Autodesk Inventor part; units mm, degrees
(part 3 of 3)
  line L321 (6.6942, 97.0319) -> (-7.3058, 97.0327) projected
  line L322 (16.4442, 97.0314) -> (16.445, 110.9522) projected
  line L323 (16.445, 110.9522) -> (30.445, 110.9515) projected
  line L324 (30.445, 110.9515) -> (30.4442, 97.0307) projected
  line L325 (30.4442, 97.0307) -> (16.4442, 97.0314) projected
  line L326 (6.9432, 78.1394) -> (6.944, 92.0602) projected
  line L327 (6.944, 92.0602) -> (20.944, 92.0594) projected
  line L328 (20.944, 92.0594) -> (20.9432, 78.1386) projected
  line L329 (20.9432, 78.1386) -> (6.9432, 78.1394) projected
  line L330 (11.6922, 59.2466) -> (11.693, 73.1674) projected
  line L331 (11.693, 73.1674) -> (25.693, 73.1667) projected
  line L332 (25.693, 73.1667) -> (25.6922, 59.2458) projected
  line L333 (25.6922, 59.2458) -> (11.6922, 59.2466) projected
  line L334 (14.0662, 40.3539) -> (14.067, 54.2747) projected
  line L335 (14.067, 54.2747) -> (28.067, 54.274) projected
  line L336 (28.067, 54.274) -> (28.0662, 40.3532) projected
  line L337 (28.0662, 40.3532) -> (14.0662, 40.3539) projected
  line L338 (-209.1848, 21.4733) -> (-209.1841, 35.3941) projected
  line L339 (-209.1841, 35.3941) -> (-195.1841, 35.3934) projected
  line L340 (-195.1841, 35.3934) -> (-195.1848, 21.4726) projected
  line L341 (-195.1848, 21.4726) -> (-209.1848, 21.4733) projected
  line L342 (-190.1848, 21.4723) -> (-190.1841, 35.3931) projected
  line L343 (-190.1841, 35.3931) -> (-176.1841, 35.3924) projected
  line L344 (-176.1841, 35.3924) -> (-176.1848, 21.4716) projected
  line L345 (-176.1848, 21.4716) -> (-190.1848, 21.4723) projected
  line L346 (-171.1848, 21.4713) -> (-171.1841, 35.3921) projected
  line L347 (-171.1841, 35.3921) -> (-157.1841, 35.3914) projected
  line L348 (-157.1841, 35.3914) -> (-157.1848, 21.4705) projected
  line L349 (-157.1848, 21.4705) -> (-171.1848, 21.4713) projected
  line L350 (-152.1848, 21.4703) -> (-152.1841, 35.3911) projected
  line L351 (-152.1841, 35.3911) -> (-138.1841, 35.3903) projected
  line L352 (-138.1841, 35.3903) -> (-138.1848, 21.4695) projected
  line L353 (-138.1848, 21.4695) -> (-152.1848, 21.4703) projected
  line L354 (-133.1848, 21.4693) -> (-133.1841, 35.3901) projected
  line L355 (-133.1841, 35.3901) -> (-119.1841, 35.3893) projected
  line L356 (-119.1841, 35.3893) -> (-119.1848, 21.4685) projected
  line L357 (-119.1848, 21.4685) -> (-133.1848, 21.4693) projected
  line L358 (-114.1848, 21.4682) -> (-114.1841, 35.3891) projected
  line L359 (-114.1841, 35.3891) -> (-100.1841, 35.3883) projected
  line L360 (-100.1841, 35.3883) -> (-100.1848, 21.4675) projected
  line L361 (-100.1848, 21.4675) -> (-114.1848, 21.4682) projected
  line L362 (-95.1848, 21.4672) -> (-95.1841, 35.388) projected
  line L363 (-95.1841, 35.388) -> (-81.1841, 35.3873) projected
  line L364 (-81.1841, 35.3873) -> (-81.1848, 21.4665) projected
  line L365 (-81.1848, 21.4665) -> (-95.1848, 21.4672) projected
  line L366 (-76.1848, 21.4662) -> (-76.1841, 35.387) projected
  line L367 (-76.1841, 35.387) -> (-62.1841, 35.3863) projected
  line L368 (-62.1841, 35.3863) -> (-62.1848, 21.4655) projected
  line L369 (-62.1848, 21.4655) -> (-76.1848, 21.4662) projected
  line L370 (-57.1848, 21.4652) -> (-57.1841, 35.386) projected
  line L371 (-57.1841, 35.386) -> (-43.1841, 35.3853) projected
  line L372 (-43.1841, 35.3853) -> (-43.1848, 21.4645) projected
  line L373 (-43.1848, 21.4645) -> (-57.1848, 21.4652) projected
  line L374 (-38.1848, 21.4642) -> (-38.1841, 35.385) projected
  line L375 (-38.1841, 35.385) -> (-24.1841, 35.3843) projected
  line L376 (-24.1841, 35.3843) -> (-24.1848, 21.4634) projected
  line L377 (-24.1848, 21.4634) -> (-38.1848, 21.4642) projected
  line L378 (-19.1848, 21.4632) -> (-19.1841, 35.384) projected
  line L379 (-19.1841, 35.384) -> (-5.1841, 35.3832) projected
  line L380 (-5.1841, 35.3832) -> (-5.1848, 21.4624) projected
  line L381 (-5.1848, 21.4624) -> (-19.1848, 21.4632) projected
  line L382 (-0.1848, 21.4622) -> (-0.1841, 35.383) projected
  line L383 (-0.1841, 35.383) -> (13.8159, 35.3822) projected
  line L384 (13.8159, 35.3822) -> (13.8152, 21.4614) projected
  line L385 (13.8152, 21.4614) -> (-0.1848, 21.4622) projected
  line L386 (18.8152, 21.4611) -> (18.8159, 35.382) projected
  line L387 (18.8159, 35.382) -> (32.8159, 35.3812) projected
  line L388 (32.8159, 35.3812) -> (32.8152, 21.4604) projected
  line L389 (32.8152, 21.4604) -> (18.8152, 21.4611) projected
  line L390 (56.567, 54.2725) -> (56.5662, 40.3517) projected
  line L391 (56.5662, 40.3517) -> (42.5662, 40.3524) projected
  line L392 (42.5662, 40.3524) -> (42.567, 54.2732) projected
  line L393 (42.567, 54.2732) -> (56.567, 54.2725) projected
  line L394 (75.567, 54.2715) -> (75.5662, 40.3506) projected
  line L395 (75.5662, 40.3506) -> (61.5662, 40.3514) projected
  line L396 (61.5662, 40.3514) -> (61.567, 54.2722) projected
  line L397 (61.567, 54.2722) -> (75.567, 54.2715) projected
  line L398 (94.567, 54.2704) -> (94.5662, 40.3496) projected
  line L399 (94.5662, 40.3496) -> (80.5662, 40.3504) projected
  line L400 (80.5662, 40.3504) -> (80.567, 54.2712) projected
  line L401 (80.567, 54.2712) -> (94.567, 54.2704) projected
  line L402 (56.5659, 35.3799) -> (56.5652, 21.4591) projected
  line L403 (56.5652, 21.4591) -> (42.5652, 21.4599) projected
  line L404 (42.5652, 21.4599) -> (42.5659, 35.3807) projected
  line L405 (42.5659, 35.3807) -> (56.5659, 35.3799) projected
  line L406 (75.5659, 35.3789) -> (75.5652, 21.4581) projected
  line L407 (75.5652, 21.4581) -> (61.5652, 21.4589) projected
  line L408 (61.5652, 21.4589) -> (61.5659, 35.3797) projected
  line L409 (61.5659, 35.3797) -> (75.5659, 35.3789) projected
  line L410 (80.5652, 21.4578) -> (80.5659, 35.3787) projected
  line L411 (80.5659, 35.3787) -> (94.5659, 35.3779) projected
  line L412 (94.5659, 35.3779) -> (94.5652, 21.4571) projected
  line L413 (94.5652, 21.4571) -> (80.5652, 21.4578) projected
  line L414 (61.5682, 78.1365) -> (61.569, 92.0573) projected
  line L415 (61.569, 92.0573) -> (75.569, 92.0565) projected
  line L416 (75.569, 92.0565) -> (75.5682, 78.1357) projected
  line L417 (75.5682, 78.1357) -> (61.5682, 78.1365) projected
  line L418 (42.5692, 97.03) -> (42.57, 110.9508) projected
  line L419 (42.57, 110.9508) -> (56.57, 110.9501) projected
  line L420 (56.57, 110.9501) -> (56.5692, 97.0293) projected
  line L421 (56.5692, 97.0293) -> (42.5692, 97.03) projected
  line L422 (61.5692, 97.029) -> (61.57, 110.9498) projected
  line L423 (61.57, 110.9498) -> (75.57, 110.9491) projected
  line L424 (75.57, 110.9491) -> (75.5692, 97.0282) projected
  line L425 (75.5692, 97.0282) -> (61.5692, 97.029) projected
  line L426 (80.5692, 97.028) -> (80.57, 110.9488) projected
  line L427 (80.57, 110.9488) -> (94.57, 110.948) projected
  line L428 (94.57, 110.948) -> (94.5692, 97.0272) projected
  line L429 (94.5692, 97.0272) -> (80.5692, 97.028) projected
  line L430 (104.3187, 87.5804) -> (104.3195, 101.5013) projected
  line L431 (104.3195, 101.5013) -> (118.3195, 101.5005) projected
  line L432 (118.3195, 101.5005) -> (118.3187, 87.5797) projected
  line L433 (118.3187, 87.5797) -> (104.3187, 87.5804) projected
  line L434 (104.3167, 49.7954) -> (104.3175, 63.7162) projected
  line L435 (104.3175, 63.7162) -> (118.3175, 63.7154) projected
  line L436 (118.3175, 63.7154) -> (118.3167, 49.7946) projected
  line L437 (118.3167, 49.7946) -> (104.3167, 49.7954) projected
  line L438 (104.3152, 21.4566) -> (104.3159, 35.3774) projected
  line L439 (104.3159, 35.3774) -> (118.3159, 35.3766) projected
  line L440 (118.3159, 35.3766) -> (118.3152, 21.4558) projected
  line L441 (118.3152, 21.4558) -> (104.3152, 21.4566) projected
  line L442 (137.3192, 97.0249) -> (123.3192, 97.0257) projected
  line L443 (123.3192, 97.0257) -> (123.32, 110.9465) projected
  line L444 (123.32, 110.9465) -> (137.32, 110.9458) projected
  line L445 (137.32, 110.9458) -> (137.3192, 97.0249) projected
  line L446 (156.3192, 97.0239) -> (142.3192, 97.0247) projected
  line L447 (142.3192, 97.0247) -> (142.32, 110.9455) projected
  line L448 (142.32, 110.9455) -> (156.32, 110.9447) projected
  line L449 (156.32, 110.9447) -> (156.3192, 97.0239) projected
  line L450 (175.3192, 97.0229) -> (161.3192, 97.0237) projected
  line L451 (161.3192, 97.0237) -> (161.32, 110.9445) projected
  line L452 (161.32, 110.9445) -> (175.32, 110.9437) projected
  line L453 (175.32, 110.9437) -> (175.3192, 97.0229) projected
  line L454 (137.3182, 78.1324) -> (123.3182, 78.1332) projected
  line L455 (123.3182, 78.1332) -> (123.319, 92.054) projected
  line L456 (123.319, 92.054) -> (137.319, 92.0532) projected
  line L457 (137.319, 92.0532) -> (137.3182, 78.1324) projected
  line L458 (156.3182, 78.1314) -> (142.3182, 78.1321) projected
  line L459 (142.3182, 78.1321) -> (142.319, 92.053) projected
  line L460 (142.319, 92.053) -> (156.319, 92.0522) projected
  line L461 (156.319, 92.0522) -> (156.3182, 78.1314) projected
  line L462 (175.3182, 78.1304) -> (161.3182, 78.1311) projected
  line L463 (161.3182, 78.1311) -> (161.319, 92.0519) projected
  line L464 (161.319, 92.0519) -> (175.319, 92.0512) projected
  line L465 (175.319, 92.0512) -> (175.3182, 78.1304) projected
  line L466 (137.3172, 59.2399) -> (123.3172, 59.2406) projected
  line L467 (123.3172, 59.2406) -> (123.318, 73.1614) projected
  line L468 (123.318, 73.1614) -> (137.318, 73.1607) projected
  line L469 (137.318, 73.1607) -> (137.3172, 59.2399) projected
  line L470 (156.3172, 59.2389) -> (142.3172, 59.2396) projected
  line L471 (142.3172, 59.2396) -> (142.318, 73.1604) projected
  line L472 (142.318, 73.1604) -> (156.318, 73.1597) projected
  line L473 (156.318, 73.1597) -> (156.3172, 59.2389) projected
  line L474 (175.3172, 59.2379) -> (161.3172, 59.2386) projected
  line L475 (161.3172, 59.2386) -> (161.318, 73.1594) projected
  line L476 (161.318, 73.1594) -> (175.318, 73.1587) projected
  line L477 (175.318, 73.1587) -> (175.3172, 59.2379) projected
  line L478 (137.3162, 40.3474) -> (123.3162, 40.3481) projected
  line L479 (123.3162, 40.3481) -> (123.317, 54.2689) projected
  line L480 (123.317, 54.2689) -> (137.317, 54.2682) projected
  line L481 (137.317, 54.2682) -> (137.3162, 40.3474) projected
  line L482 (156.3162, 40.3463) -> (142.3162, 40.3471) projected
  line L483 (142.3162, 40.3471) -> (142.317, 54.2679) projected
  line L484 (142.317, 54.2679) -> (156.317, 54.2671) projected
  line L485 (156.317, 54.2671) -> (156.3162, 40.3463) projected
  line L486 (175.3162, 40.3453) -> (161.3162, 40.3461) projected
  line L487 (161.3162, 40.3461) -> (161.317, 54.2669) projected
  line L488 (161.317, 54.2669) -> (175.317, 54.2661) projected
  line L489 (175.317, 54.2661) -> (175.3162, 40.3453) projected
  line L490 (137.3152, 21.4548) -> (123.3152, 21.4556) projected
  line L491 (123.3152, 21.4556) -> (123.3159, 35.3764) projected
  line L492 (123.3159, 35.3764) -> (137.3159, 35.3756) projected
  line L493 (137.3159, 35.3756) -> (137.3152, 21.4548) projected
  line L494 (156.3152, 21.4538) -> (142.3152, 21.4546) projected
  line L495 (142.3152, 21.4546) -> (142.3159, 35.3754) projected
  line L496 (142.3159, 35.3754) -> (156.3159, 35.3746) projected
  line L497 (156.3159, 35.3746) -> (156.3152, 21.4538) projected
  line L498 (161.3152, 21.4535) -> (161.3159, 35.3743) projected
  line L499 (161.3159, 35.3743) -> (175.3159, 35.3736) projected
  line L500 (175.3159, 35.3736) -> (175.3152, 21.4528) projected
  line L501 (175.3152, 21.4528) -> (161.3152, 21.4535) projected
  line L502 (-247.1863, -6.8635) -> (-247.1856, 7.0574) projected
  line L503 (-247.1856, 7.0574) -> (-233.1856, 7.0566) projected
  line L504 (-233.1856, 7.0566) -> (-233.1863, -6.8642) projected
  line L505 (-233.1863, -6.8642) -> (-247.1863, -6.8635) projected
  line L506 (-228.1863, -6.8645) -> (-228.1856, 7.0563) projected
  line L507 (-228.1856, 7.0563) -> (-214.1856, 7.0556) projected
  line L508 (-214.1856, 7.0556) -> (-214.1863, -6.8652) projected
  line L509 (-214.1863, -6.8652) -> (-228.1863, -6.8645) projected
  line L510 (-209.1863, -6.8655) -> (-209.1856, 7.0553) projected
  line L511 (-209.1856, 7.0553) -> (-195.1856, 7.0546) projected
  line L512 (-195.1856, 7.0546) -> (-195.1863, -6.8662) projected
  line L513 (-195.1863, -6.8662) -> (-209.1863, -6.8655) projected
  line L514 (-190.1863, -6.8665) -> (-190.1856, 7.0543) projected
  line L515 (-190.1856, 7.0543) -> (-176.1856, 7.0536) projected
  line L516 (-176.1856, 7.0536) -> (-176.1863, -6.8672) projected
  line L517 (-176.1863, -6.8672) -> (-190.1863, -6.8665) projected
  line L518 (-161.6863, -6.868) -> (-161.6856, 7.0528) projected
  line L519 (-161.6856, 7.0528) -> (-147.6856, 7.052) projected
  line L520 (-147.6856, 7.052) -> (-147.6863, -6.8688) projected
  line L521 (-147.6863, -6.8688) -> (-161.6863, -6.868) projected
  line L522 (-142.6863, -6.869) -> (-142.6856, 7.0518) projected
  line L523 (-142.6856, 7.0518) -> (-128.6856, 7.051) projected
  line L524 (-128.6856, 7.051) -> (-128.6863, -6.8698) projected
  line L525 (-128.6863, -6.8698) -> (-142.6863, -6.869) projected
  line L526 (-123.6863, -6.87) -> (-123.6856, 7.0508) projected
  line L527 (-123.6856, 7.0508) -> (-109.6856, 7.05) projected
  line L528 (-109.6856, 7.05) -> (-109.6863, -6.8708) projected
  line L529 (-109.6863, -6.8708) -> (-123.6863, -6.87) projected
  line L530 (-104.6863, -6.8711) -> (-104.6856, 7.0498) projected
  line L531 (-104.6856, 7.0498) -> (-90.6856, 7.049) projected
  line L532 (-90.6856, 7.049) -> (-90.6863, -6.8718) projected
  line L533 (-90.6863, -6.8718) -> (-104.6863, -6.8711) projected
  line L534 (-76.1863, -6.8726) -> (-76.1856, 7.0482) projected
  line L535 (-76.1856, 7.0482) -> (-62.1856, 7.0475) projected
  line L536 (-62.1856, 7.0475) -> (-62.1863, -6.8733) projected
  line L537 (-62.1863, -6.8733) -> (-76.1863, -6.8726) projected
  line L538 (-57.1863, -6.8736) -> (-57.1856, 7.0472) projected
  line L539 (-57.1856, 7.0472) -> (-43.1856, 7.0465) projected
  line L540 (-43.1856, 7.0465) -> (-43.1863, -6.8743) projected
  line L541 (-43.1863, -6.8743) -> (-57.1863, -6.8736) projected
  line L542 (-38.1863, -6.8746) -> (-38.1856, 7.0462) projected
  line L543 (-38.1856, 7.0462) -> (-24.1856, 7.0455) projected
  line L544 (-24.1856, 7.0455) -> (-24.1863, -6.8754) projected
  line L545 (-24.1863, -6.8754) -> (-38.1863, -6.8746) projected
  line L546 (-19.1863, -6.8756) -> (-19.1856, 7.0452) projected
  line L547 (-19.1856, 7.0452) -> (-5.1856, 7.0444) projected
  line L548 (-5.1856, 7.0444) -> (-5.1863, -6.8764) projected
  line L549 (-5.1863, -6.8764) -> (-19.1863, -6.8756) projected
  line L550 (18.8137, -6.8777) -> (18.8144, 7.0432) projected
  line L551 (18.8144, 7.0432) -> (32.8144, 7.0424) projected
  line L552 (32.8144, 7.0424) -> (32.8137, -6.8784) projected
  line L553 (32.8137, -6.8784) -> (18.8137, -6.8777) projected
  line L554 (-252.0614, -9.3491) -> (180.1886, -9.3721) projected
  ellipse E814 centre (180.1888, -4.649) end of major axis (184.9388, -4.6493) minor radius 4.7231 (180.1886, -9.3721) -> (184.9388, -4.6493) ccw projected
  line L555 (184.9388, -4.6493) -> (184.9449, 108.7059) projected
  ellipse E815 centre (180.1949, 108.7062) end of major axis (184.9449, 108.7059) minor radius 4.7231 (184.9449, 108.7059) -> (180.1951, 113.4293) ccw projected
  line L556 (180.1951, 113.4293) -> (-252.0549, 113.4524) projected
  ellipse E816 centre (-252.0551, 108.7293) end of major axis (-256.8051, 108.7295) minor radius 4.7231 (-252.0549, 113.4524) -> (-256.8051, 108.7295) ccw projected
  line L557 (-256.8051, 108.7295) -> (-256.8112, -4.6257) projected
  ellipse E817 centre (-252.0612, -4.6259) end of major axis (-256.8112, -4.6257) minor radius 4.7231 (-256.8112, -4.6257) -> (-252.0614, -9.3491) ccw projected
  line L558 (180.1884, -12.9036) -> (-252.0616, -12.8805)
  line L559 (-259.8112, -5.157) -> (-259.8052, 108.1982)
  line L560 (-252.0548, 115.921) -> (180.1952, 115.8979)
  line L561 (187.9449, 108.1743) -> (187.9388, -5.1809)
  line L562 (187.9449, 108.7058) -> (187.9388, -4.6494)
  line L563 (180.1884, -12.3722) -> (-252.0616, -12.3491)
  line L564 (-259.8112, -4.6255) -> (-259.8052, 108.7297)
  line L565 (-252.0547, 116.4524) -> (180.1953, 116.4294)
  ellipse E818 centre (-168.9362, -4.6304) end of major axis (-167.5862, -4.6304) minor radius 1.3424 projected
  ellipse E819 centre (-223.5588, 40.2423) end of major axis (-222.2088, 40.2423) minor radius 1.3424 projected
  ellipse E820 centre (-202.181, 92.1956) end of major axis (-200.831, 92.1956) minor radius 1.3424 projected
  ellipse E821 centre (-145.1839, 38.6323) end of major axis (-143.8339, 38.6322) minor radius 1.3424 projected
  ellipse E822 centre (-111.9319, 74.9996) end of major axis (-110.5819, 74.9995) minor radius 1.3424 projected
  ellipse E823 centre (-69.1839, 38.6282) end of major axis (-67.8339, 38.6281) minor radius 1.3424 projected
  ellipse E824 centre (139.8181, 75.6464) end of major axis (141.1681, 75.6464) minor radius 1.3424 projected
  ellipse E825 centre (139.8161, 37.8614) end of major axis (141.1661, 37.8613) minor radius 1.3424 projected
  ellipse E826 centre (78.0661, 37.8647) end of major axis (79.4161, 37.8646) minor radius 1.3424 projected
  ellipse E827 centre (-83.4362, -4.6349) end of major axis (-82.0862, -4.635) minor radius 1.3424 projected
  ellipse E828 centre (-26.4319, 76.2579) end of major axis (-25.0819, 76.2578) minor radius 1.3424 projected
  ellipse E829 centre (37.6888, -4.6414) end of major axis (39.0388, -4.6415) minor radius 1.3424 projected
  ellipse E830 centre (9.1912, 40.2299) end of major axis (10.5412, 40.2298) minor radius 1.3424 projected
  ellipse E831 centre (30.5678, 70.9291) end of major axis (31.9178, 70.9291) minor radius 1.3424 projected
  ellipse E832 centre (180.1918, 52.0286) end of major axis (181.5418, 52.0285) minor radius 1.3424 projected
  ellipse E833 centre (180.1888, -4.649) end of major axis (181.5388, -4.6491) minor radius 1.3424 projected
  ellipse E834 centre (180.1949, 108.7062) end of major axis (181.5449, 108.7061) minor radius 1.3424 projected
  ellipse E835 centre (11.5699, 108.7152) end of major axis (12.9199, 108.7151) minor radius 1.3424 projected
  ellipse E836 centre (97.8229, 108.7106) end of major axis (99.1729, 108.7105) minor radius 1.3424 projected
  ellipse E837 centre (-59.6801, 108.719) end of major axis (-58.3301, 108.7189) minor radius 1.3424 projected
  ellipse E838 centre (-154.6801, 108.7241) end of major axis (-153.3301, 108.724) minor radius 1.3424 projected
  ellipse E839 centre (-252.0551, 108.7293) end of major axis (-250.7051, 108.7292) minor radius 1.3424 projected
  ellipse E840 centre (-252.0582, 52.0517) end of major axis (-250.7082, 52.0516) minor radius 1.3424 projected
  ellipse E841 centre (-252.0612, -4.6259) end of major axis (-250.7112, -4.626) minor radius 1.3424 projected
  spline S0 degree 5 poles (187.9388, -5.1809) (187.9388, -6.3965) (187.6987, -7.6121) (187.2184, -8.7644) (185.8312, -10.8164) (183.7714, -12.192) (182.6182, -12.6665) (181.4033, -12.9037) (180.1884, -12.9036) knots 0 0 0 0 0 0 0.500148 0.500148 0.500148 1 1 1 1 1 1
  spline S1 degree 5 poles (-252.0616, -12.8805) (-253.2765, -12.8805) (-254.4914, -12.6432) (-255.6446, -12.1685) (-257.7043, -10.7928) (-259.0913, -8.7406) (-259.5714, -7.5882) (-259.8113, -6.3726) (-259.8113, -5.157) knots 0 0 0 0 0 0 0.499852 0.499852 0.499852 1 1 1 1 1 1
  spline S2 degree 5 poles (-259.8052, 108.1982) (-259.8052, 109.4139) (-259.565, 110.6295) (-259.0848, 111.7818) (-257.6976, 113.8338) (-255.6378, 115.2094) (-254.4846, 115.6839) (-253.2697, 115.9211) (-252.0548, 115.921) knots 0 0 0 0 0 0 0.500148 0.500148 0.500148 1 1 1 1 1 1
  spline S3 degree 5 poles (180.1952, 115.8979) (181.4101, 115.8979) (182.625, 115.6605) (183.7782, 115.1859) (185.8379, 113.8101) (187.2249, 111.758) (187.705, 110.6056) (187.945, 109.39) (187.9449, 108.1743) knots 0 0 0 0 0 0 0.499852 0.499852 0.499852 1 1 1 1 1 1
  spline S4 degree 5 poles (180.1953, 116.4294) (181.4102, 116.4293) (182.6251, 116.192) (183.7782, 115.7174) (185.8379, 114.3416) (187.2249, 112.2895) (187.705, 111.137) (187.945, 109.9214) (187.9449, 108.7058) knots 0 0 0 0 0 0 0.499852 0.499852 0.499852 1 1 1 1 1 1
  spline S5 degree 5 poles (187.9388, -4.6494) (187.9388, -5.865) (187.6987, -7.0806) (187.2185, -8.233) (185.8312, -10.285) (183.7714, -11.6605) (182.6182, -12.135) (181.4033, -12.3722) (180.1884, -12.3722) knots 0 0 0 0 0 0 0.500148 0.500148 0.500148 1 1 1 1 1 1
  spline S6 degree 5 poles (-252.0616, -12.3491) (-253.2765, -12.349) (-254.4914, -12.1117) (-255.6445, -11.6371) (-257.7042, -10.2613) (-259.0912, -8.2092) (-259.5713, -7.0568) (-259.8113, -5.8411) (-259.8112, -4.6255) knots 0 0 0 0 0 0 0.499852 0.499852 0.499852 1 1 1 1 1 1
  spline S7 degree 5 poles (-259.8052, 108.7297) (-259.8051, 109.9453) (-259.565, 111.1609) (-259.0848, 112.3133) (-257.6976, 114.3653) (-255.6377, 115.7408) (-254.4845, 116.2153) (-253.2696, 116.4525) (-252.0547, 116.4524) knots 0 0 0 0 0 0 0.500148 0.500148 0.500148 1 1 1 1 1 1
  point P0 (-46.4829, -23.1847)
  dimension "d0" = 3
  dimension "d1" = 3
  constraints: 16 end point, 14 parallel, 866 other
ref_plane "Work Plane2" through (-253.3416, -140.7462, 28.9028) normal (0, 0, 1) x (1, 0, 0)
extrude "Extrusion1" add sketch "Sketch1" along normal up to surface contours L558 S1 L559 S6 L563 S5 L561 S0 | S5 L563 S6 L559 S2 L560 S3 L561 | S3 L560 S2 L564 S7 L565 S4 L562 surface through (-253.3416, -140.7462, 28.9028) normal (0, 0, 1)
sketch "Sketch2" plane through (-46.4829, -22.3295, 9.2415) normal (0, 0.1062088, 0.9943439) x (-1, 0, 0)
  line L0 (-256.8051, 108.7295) -> (-256.8112, -5.1571) projected
  ellipse E0 centre (-252.0612, -5.1574) end of major axis (-256.8112, -5.1571) minor radius 4.7231 (-256.8112, -5.1571) -> (-252.0615, -9.8805) ccw projected
  line L1 (-252.0615, -9.8805) -> (180.1885, -9.9036) projected
  ellipse E1 centre (180.1888, -5.1804) end of major axis (175.4388, -5.1802) minor radius 4.7231 (180.1885, -9.9036) -> (184.9388, -5.1807) ccw projected
  line L2 (184.9388, -5.1807) -> (184.9449, 108.7059) projected
  ellipse E2 centre (180.1949, 108.7062) end of major axis (184.9449, 108.7059) minor radius 4.7231 (184.9449, 108.7059) -> (180.1951, 113.4293) ccw projected
  line L3 (180.1951, 113.4293) -> (-252.0549, 113.4524) projected
  ellipse E3 centre (-252.0551, 108.7293) end of major axis (-256.8051, 108.7295) minor radius 4.7231 (-252.0549, 113.4524) -> (-256.8051, 108.7295) ccw projected
  line L4 (187.9449, 108.7058) -> (187.9388, -5.1809) projected
  spline S0 degree 5 poles (187.9388, -5.1809) (187.9388, -6.3965) (187.6987, -7.6121) (187.2184, -8.7644) (185.8312, -10.8164) (183.7714, -12.192) (182.6182, -12.6665) (181.4033, -12.9037) (180.1884, -12.9036) knots 0 0 0 0 0 0 0.500148 0.500148 0.500148 1 1 1 1 1 1 projected
  line L5 (180.1884, -12.9036) -> (-252.0616, -12.8805) projected
  spline S1 degree 5 poles (-252.0616, -12.8805) (-253.2765, -12.8805) (-254.4914, -12.6432) (-255.6446, -12.1685) (-257.7043, -10.7928) (-259.0913, -8.7406) (-259.5714, -7.5882) (-259.8113, -6.3726) (-259.8113, -5.157) knots 0 0 0 0 0 0 0.499852 0.499852 0.499852 1 1 1 1 1 1 projected
  line L6 (-259.8112, -5.157) -> (-259.8052, 108.7297) projected
  spline S2 degree 5 poles (-259.8052, 108.7297) (-259.8051, 109.9453) (-259.565, 111.1609) (-259.0848, 112.3133) (-257.6976, 114.3653) (-255.6377, 115.7408) (-254.4845, 116.2153) (-253.2696, 116.4525) (-252.0547, 116.4524) knots 0 0 0 0 0 0 0.500148 0.500148 0.500148 1 1 1 1 1 1 projected
  line L7 (-252.0547, 116.4524) -> (180.1953, 116.4294) projected
  spline S3 degree 5 poles (180.1953, 116.4294) (181.4102, 116.4293) (182.6251, 116.192) (183.7782, 115.7174) (185.8379, 114.3416) (187.2249, 112.2895) (187.705, 111.137) (187.945, 109.9214) (187.9449, 108.7058) knots 0 0 0 0 0 0 0.499852 0.499852 0.499852 1 1 1 1 1 1 projected
  point P0 (-46.4829, -23.1847)
  constraints: 8 other
extrude "Extrusion2" add sketch "Sketch2" against normal blind 3 contours E3 L3 E2 L2 E1 L1 E0 L0 | L4 S0 L5 S1 L6 S2 L7 S3
body "Solid1"
